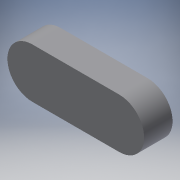
# Autodesk Inventor part: Joint
Saved by Autodesk Inventor 2018 (Build 220105000, 105)
## iProperties
Created: 2004-11-28
Document SubType Name: Modeling
Designer: Autodesk, Inc.
Manufacturer: Standard
Standards Organization: Custom
Description: SWING ARM, JOINT
Mass: 127.24 g
Surface Area: 175.174 cm^2
Volume: 127.24 cm^3
Density: 1 g/cm^3
Material: Generic
Appearance: Default
CAGE: 1LJX3
Dept. ID: Product Design
Description #2: ---
Finish #1: ---
Finish #2: ---
Material ID: ---
Project Number: ---
Author: Autodesk, Inc.
Autodesk Inventor part; units mm, degrees
ref_plane "YZ Plane" through (0, 0, 0) normal (1, 0, 0) x (0, 1, 0)
ref_plane "XZ Plane" through (0, 0, 0) normal (0, 1, 0) x (-1, 0, 0)
ref_plane "XY Plane" through (0, 0, 0) normal (0, 0, 1) x (1, 0, 0)
sketch "Sketch1" plane through (0, 0, 0) normal (0, 0, 1) x (1, 0, 0)
  line L0 (-38.8938, 22.225) -> (38.8937, 22.225)
  line L1 (38.8937, 22.225) -> (38.8938, -22.225)
  line L2 (38.8938, -22.225) -> (-38.8937, -22.225)
  line L3 (-38.8937, -22.225) -> (-38.8938, 22.225)
  circle A0 centre (-38.8938, 0) radius 22.225
  circle A1 centre (38.8938, 0) radius 22.225
  point P0 (0, 0)
  point P1 (0, -22.225)
  dimension "d0" = 44.45
  dimension "d1" = 77.7875
  constraints: 8 end point, 3 midpoint, 2 parallel, 2 vertical alignment, 1 centre point, 1 horizontal, 1 horizontal alignment, 1 perpendicular, 1 tangent, 2 other
  measures "d0" distance of L0.end L1.end
  measures "d1" distance of L0.start L0.end
extrude "Extrusion1" add sketch "Sketch1" along normal mid plane 25.4
body "Solid1"
